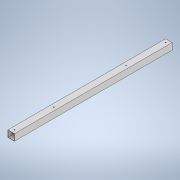
# Autodesk Inventor part: 24 in 1x1 for drive
Saved by Autodesk Inventor 2020 (Build 240168000, 168)
## iProperties
Created: 2020-01-14
Part Number: 24 in 1x1 for drive
Material: Generic
Document SubType Name: Modeling
Designer: aidan
Density: 1 g/cm^3
Appearance: Default
Author: aidan
Autodesk Inventor part; units mm, degrees
ref_plane "YZ Plane" through (0, 0, 0) normal (1, 0, 0) x (0, 1, 0)
ref_plane "XZ Plane" through (0, 0, 0) normal (0, 1, 0) x (-1, 0, 0)
ref_plane "XY Plane" through (0, 0, 0) normal (0, 0, 1) x (1, 0, 0)
sketch "Sketch1" plane through (0, 0, 0) normal (0, 0, 1) x (1, 0, 0)
  line L0 (-14.0074, 10.2243) -> (11.3926, 10.2243)
  line L1 (11.3926, 10.2243) -> (11.3926, -15.1757)
  line L2 (11.3926, -15.1757) -> (-14.0074, -15.1757)
  line L3 (-14.0074, -15.1757) -> (-14.0074, 10.2243)
  line L4 (10.1226, 8.9543) -> (-12.7374, 8.9543)
  line L5 (-12.7374, 8.9543) -> (-12.7374, -13.9057)
  line L6 (-12.7374, -13.9057) -> (10.1226, -13.9057)
  line L7 (10.1226, -13.9057) -> (10.1226, 8.9543)
  point P0 (0, 0)
  dimension "d0" = 25.4
  dimension "d1" = 1.27
  constraints: 16 end point, 4 parallel, 3 perpendicular, 1 horizontal, 3 other
  measures "d0" distance of L0.start L0.end
  measures "d1" distance between parallel lines of L0 L4
extrude "Extrusion2" add sketch "Sketch1" along normal blind 609.6
sketch "Sketch2" plane through (-14.0074, 10.2243, 0) normal (0, 1, 0) x (1, 0, 0)
  circle A0 centre (12.7, -165.1) radius 1.7272
  circle A1 centre (12.7, -444.5) radius 1.7272
  circle A2 centre (12.7, -596.9) radius 1.7272
  circle A3 centre (12.7, -12.7) radius 1.7272
  line L0 (12.7, -275.2188) -> (12.7, -289.6377) construction
  line L1 (25.4, -609.6) -> (0, -609.6) projected
  line L2 (25.4, 0) -> (25.4, -609.6) projected
  line L3 (25.4, 0) -> (0, 0) projected
  point P0 (14.0074, 0)
  dimension "d6" = 3.4544
  dimension "d7" = 12.7
  dimension "d8" = 12.7
  dimension "d9" = 12.7
  dimension "d11" = 152.4
  dimension "d15" = 152.4
  constraints: 4 centre point, 4 point on line, 3 equal radius, 2 end point, 1 vertical
  measures "d6" diameter of A2
  measures "d7" distance from line of A2.centre L1
  measures "d8" distance between parallel lines of L2 L0
  measures "d9" distance from line of L3 A3.centre
  measures "d11" distance of A1.centre A2.centre
  measures "d15" distance of A3.centre A0.centre
extrude "Extrusion3" cut sketch "Sketch2" against normal through all
equation "\"d4\" = d2"
equation "\"d11\" = d14"
equation "\"d15\" = d14"
equation "\"d2\" = 609.6"
equation "\"d14\" = 152.4"
body "Solid2"
